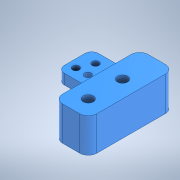
# Autodesk Inventor part: CableChain_Mount
Saved by Autodesk Inventor 2021 (Build 250183000, 183)
## iProperties
Created: 2021-12-15
Part Number: CableChain_Mount
Material: Generic
Document SubType Name: Modeling
Designer: Jorian Brusind
Density: 1 g/cm^3
Appearance: Cyan
Author: Jorian Brusind
Autodesk Inventor part; units mm, degrees
ref_plane "YZ Plane" through (0, 0, 0) normal (1, 0, 0) x (0, 1, 0)
ref_plane "XZ Plane" through (0, 0, 0) normal (0, 1, 0) x (-1, 0, 0)
ref_plane "XY Plane" through (0, 0, 0) normal (0, 0, 1) x (1, 0, 0)
sketch "Sketch1" plane through (0, 0, 0) normal (0, 1, 0) x (-1, 0, 0)
  line L0 (0, 0) -> (20, 0)
  line L1 (20, 0) -> (20, -50)
  line L2 (20, -50) -> (0, -50)
  line L3 (0, -50) -> (0, 0)
  line L4 (0, -50) -> (48, -50)
  line L5 (48, -50) -> (48, -30)
  line L6 (48, -30) -> (0, -30)
  line L7 (0, -30) -> (0, -50)
  circle A0 centre (10, -10) radius 3
  circle A1 centre (10, -30) radius 3
  line L8 (20, -50) -> (20, -36)
  line L9 (20, -36) -> (31, -36)
  line L10 (31, -36) -> (36.25, -36)
  circle A2 centre (36.25, -36) radius 2
  line L11 (36.25, -36) -> (43.25, -36)
  circle A3 centre (43.25, -36) radius 2
  line L12 (39.75, -36) -> (39.75, -44)
  circle A4 centre (39.75, -44) radius 2
  point P0 (20, -30)
  dimension "d0" = 20
  dimension "d1" = 50
  dimension "d2" = 48
  dimension "d3" = 20
  dimension "d4" = 6
  dimension "d5" = 6
  dimension "d6" = 10
  dimension "d7" = 10
  dimension "d8" = 20
  dimension "d9" = 10
  dimension "d10" = 11
  dimension "d11" = 5.25
  dimension "d12" = 14
  dimension "d13" = 4
  dimension "d14" = 7
  dimension "d15" = 4
  dimension "d21" = 8
  dimension "d22" = 4
  constraints: 26 end point, 5 centre point, 4 horizontal, 4 parallel, 3 coincident, 3 perpendicular, 1 midpoint, 1 point on line, 1 vertical
  measures "d0" distance of L1.end L2.end
  measures "d1" distance of L0.end L1.end
  measures "d2" distance of L6.end L5.end
  measures "d3" distance of L5.end L4.end
  measures "d4" diameter of A0
  measures "d5" diameter of A1
  measures "d6" distance from line of L0 A0.centre
  measures "d7" distance from line of L1 A0.centre
  measures "d8" distance of A0.centre A1.centre
  measures "d9" distance from line of L1 A1.centre
  measures "d10" distance of L8.end L9.end
  measures "d11" distance of L9.end L10.end
  measures "d12" distance between parallel lines of L4 L9
  measures "d13" diameter of A2
  measures "d14" distance of L11.start L11.end
  measures "d15" diameter of A3
  measures "d21" distance of L12.start L12.end
  measures "d22" diameter of A4
extrude "Extrusion1" add sketch "Sketch1" along normal blind 6 contours L0 L1 L6 A1 L3 | L6 A1 L1 L2 L3 | L6 L5 L4 L1
fillet "Fillet1" radius 4 6 edges at (-20, 3, 0) (0, 3, 0) (-20, 3, -30) (-48, 3, -30) (-48, 3, -50) (0, 3, -50)
sketch "Sketch2" plane through (0, 6, 0) normal (0, 1, 0) x (1, 0, 0)
  line L0 (0, 0) -> (-20, 0)
  line L1 (-20, 0) -> (-20, 50)
  line L2 (-20, 50) -> (0, 50)
  line L3 (0, 50) -> (0, 0)
  circle A0 centre (-10, 30) radius 3 projected
  circle A1 centre (-10, 30) radius 3
  circle A2 centre (-10, 10) radius 3 projected
  circle A3 centre (-10, 10) radius 3
  dimension "d23" = 20
  dimension "d24" = 50
  constraints: 8 end point, 2 centre point, 2 coincident, 2 parallel, 1 horizontal, 1 perpendicular
  measures "d23" distance of L1.end L2.end
  measures "d24" distance of L0.end L1.end
extrude "Extrusion2" add sketch "Sketch2" along normal blind 14
fillet "Fillet2" radius 5 3 edges at (0, 13, -50) (0, 13, 0) (-20, 13, 0)
fillet "Fillet3" radius 5 1 edges at (-20, 13, -50)
body "Solid1"
